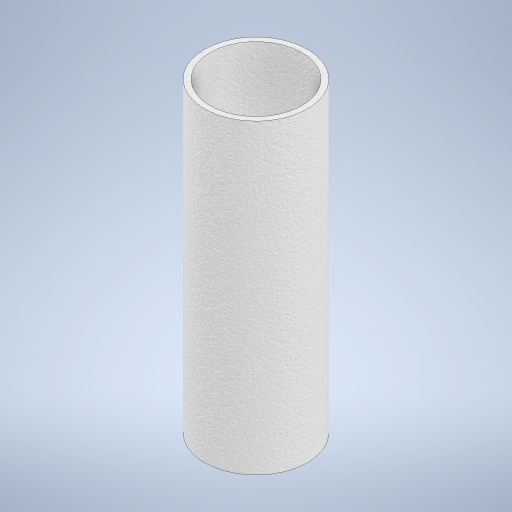
# Autodesk Inventor part: Solid_electrolyte
Saved by Autodesk Inventor 2023 (Build 270158000, 158)
## iProperties
Created: 2022-09-20
Part Number: Solid_electrolyte
Material: Бетон, легкий
Document SubType Name: Modeling
Designer: Makar
Density: 3.95 g/cm^3
Appearance: С грубой текстурой — белый
Mass: 95.5515 g
Surface Area: 246.301 cm^2
Volume: 24.1903 cm^3
Author: Makar
Autodesk Inventor part; units mm, degrees
ref_plane "YZ Plane" through (0, 0, 0) normal (1, 0, 0) x (0, 1, 0)
ref_plane "XZ Plane" through (0, 0, 0) normal (0, 1, 0) x (-1, 0, 0)
ref_plane "XY Plane" through (0, 0, 0) normal (0, 0, 1) x (1, 0, 0)
sketch "Эскиз1" plane through (0, 0, 0) normal (0, 1, 0) x (-1, 0, 0)
  circle A0 centre (0, 0) radius 14.5
  circle A1 centre (0, 0) radius 16.5
  circle A2 centre (0, 0) radius 18.5
  dimension "d0" = 29
  dimension "d1" = 33
  dimension "d2" = 37
  constraints: 3 centre point, 3 coincident
  measures "d0" diameter of A0
  measures "d1" diameter of A1
  measures "d2" diameter of A2
extrude "Выдавливание1" add sketch "Эскиз1" along normal blind 110 contours A2
